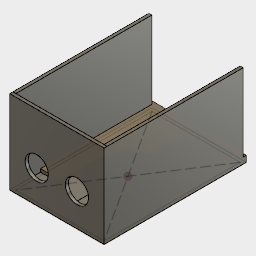
bottom shell v2 v7 (Autodesk Fusion 360 design; units mm, degrees)
Autodesk Fusion 360 part; units mm, degrees
note: some values were not read from the file. Set by a fixed rule: which sketch regions a step uses.
sketch "Sketch1" plane through (0, 0, 0) normal (0, 1, 0) x (1, 0, 0)
  line L0 (14.25, 22) -> (-14.25, 22)
  line L1 (-14.25, 22) -> (-14.25, -22)
  line L2 (-14.25, -22) -> (14.25, -22)
  line L3 (14.25, -22) -> (14.25, 22)
  line L4 (14.25, 22) -> (-14.25, -22) construction
  line L5 (-14.25, 22) -> (14.25, -22) construction
  line L6 (-15.25, 23) -> (-15.25, -23)
  line L7 (-15.25, -23) -> (15.25, -23)
  line L8 (15.25, -23) -> (15.25, 23)
  line L9 (15.25, 23) -> (-15.25, 23)
  dimension "d1" = 44
  dimension "d2" = 28.5
  dimension "d3" = 1
  measures "d1" distance of L0.end L1.end
  measures "d2" distance of L1.end L2.end
extrude "Extrude2" add sketch "Sketch1" along normal blind 2 contours L0 L1 L2 L3 makes body 1
extrude "Extrude1" add sketch "Sketch1" along normal blind 17 separate body makes body 2
sketch "Sketch2" plane through (0, 0, 23) normal (0, 0, 1) x (1, 0, 0)
  line L0 (-15.25, 0) -> (15.25, 0)
  line L1 (15.25, 0) -> (15.25, 17)
  line L2 (15.25, 17) -> (-15.25, 17)
  line L3 (-15.25, 17) -> (-15.25, 0)
  line L4 (0, 0) -> (0, 2)
  line L5 (-14.25, 2) -> (-16.75, 2)
  line L6 (14.25, 2) -> (15.25, 2)
  line L7 (14.25, 0) -> (14.25, 17)
  line L8 (-14.25, 0) -> (-14.25, 17)
  line L9 (-14.25, 2) -> (14.25, 2)
  line L10 (0, 2) -> (0, 4.8)
  line L11 (0, 4.8) -> (0, 8.55)
  line L12 (1.1168, 4.8) -> (-1, 4.8)
  line L13 (14.25, 10.55) -> (10.25, 10.55)
  line L14 (-14.25, 10.55) -> (-10.25, 10.55)
  line L15 (-10.25, 10.55) -> (-6.5, 10.55)
  line L16 (10.25, 10.55) -> (6.5, 10.55)
  circle A0 centre (-6.5, 10.55) radius 3.75
  circle A1 centre (6.5, 10.55) radius 3.75
  line L17 (0, 8.55) -> (0, 10.55)
  line L18 (-14.25, 10.55) -> (-6, 10.55)
  line L19 (14.25, 10.55) -> (6, 10.55)
  point P0 (-14.25, 2)
  point P1 (14.25, 2)
  point P2 (14.25, 0)
  point P3 (14.25, 17)
  point P4 (-14.25, 0)
  point P5 (-14.25, 17)
  dimension "d8" = 2
  dimension "d13" = 2.8
  dimension "d14" = 3.75
  dimension "d15" = 4
  dimension "d16" = 4
  dimension "d17" = 3.75
  dimension "d18" = 3.75
  dimension "d19" = 7.5
  dimension "d20" = 7.5
  dimension "d51" = 2
  measures "d8" distance of L4.start L4.end
  measures "d13" distance of L4.end L10.end
  measures "d14" distance of L10.end L11.end
  measures "d15" distance of L13.start L13.end
  measures "d16" distance of L14.start L14.end
  measures "d17" distance of L14.end L15.end
  measures "d18" distance of L13.end L16.end
  measures "d19" diameter of A0
  measures "d20" diameter of A1
  measures "d51" distance of L11.end L17.end
extrude "Extrude3" cut sketch "Sketch2" against normal blind 6 contours A0 | A1 bodies 2
sketch "Sketch3" plane through (0, 0, -23) normal (0, 0, -1) x (-1, 0, 0)
  line L0 (-15.25, 0) -> (15.25, 0)
  line L1 (15.25, 0) -> (15.25, 17)
  line L2 (15.25, 17) -> (-15.25, 17)
  line L3 (-15.25, 17) -> (-15.25, 0)
  line L4 (0, 0) -> (0, 2)
  line L5 (0, 2) -> (0, 4.8)
  line L6 (0, 4.8) -> (0, 8.55)
  circle A0 centre (0, 8.55) radius 3.75
  dimension "d23" = 2
  dimension "d24" = 2.8
  dimension "d25" = 3.75
  dimension "d26" = 7.5
  measures "d23" distance of L4.start L4.end
  measures "d24" distance of L4.end L5.end
  measures "d25" distance of L5.end L6.end
  measures "d26" diameter of A0
extrude "Extrude4" cut sketch "Sketch3" against normal blind 6 contours A0 bodies 2
sketch "Sketch4" plane through (15.25, 0, 0) normal (1, 0, 0) x (0, 0, -1)
  line L0 (-23, 0) -> (23, 0)
  line L1 (23, 0) -> (23, 17)
  line L2 (23, 17) -> (-23, 17)
  line L3 (-23, 17) -> (-23, 0)
  line L4 (-22, 0) -> (-22, 17)
  line L5 (-23, 4.2398) -> (-22, 4.2398)
  line L6 (23, 4.2398) -> (21.5, 4.2398)
  line L7 (0, 0) -> (0, 2)
  line L8 (-22, 2) -> (22, 2)
  line L9 (22, 2) -> (22, 17)
  line L10 (22, 17) -> (-22, 17)
  line L11 (-22, 17) -> (-22, 2)
  line L12 (-22, 6.4795) -> (22, 6.4795)
  line L13 (22, 6.4795) -> (22, 17)
  line L14 (22, 17) -> (-22, 17)
  line L15 (-22, 17) -> (-22, 6.4795)
  point P0 (-22, 2)
  point P1 (22, 17)
  dimension "d29" = 2
  measures "d29" distance of L7.start L7.end
extrude "Extrude5" cut sketch "Sketch4" against normal blind 71 contours L2 L4 L9 L10 L11 L12 L13 L14 L15 bodies 2
extrude "Extrude6" add 2 faces at (14.9167, 6.4795, 7.3333) (-14.5833, 6.4795, 7.3333) along direction (0, 1, 0) blind 0.02 on bodies 2 bodies 2
extrude "Extrude7" add 1 faces at (-1.71, 2.3531, 22) along direction (0, 0, -1) blind 1 on bodies 2 bodies 2 1
extrude "Extrude8" add 1 faces at (11.0278, 11.0516, -22) along direction (0, 0, 1) blind 1 on bodies 2 bodies 2
sketch "Sketch6" plane through (0, 2, 0) normal (0, 1, 0) x (-1, 0, 0)
  line L0 (-14.25, -21) -> (14.25, -21)
  line L1 (14.25, -21) -> (14.25, 21)
  line L2 (14.25, 21) -> (-14.25, 21)
  line L3 (-14.25, 21) -> (-14.25, -21)
  line L4 (-6, 7) -> (6, 7)
  line L5 (6, 7) -> (6, -7)
  line L6 (6, -7) -> (-6, -7)
  line L7 (-6, -7) -> (-6, 7)
  line L8 (-6, 7) -> (6, -7) construction
  line L9 (6, 7) -> (-6, -7) construction
extrude "Extrude9" cut sketch "Sketch6" against normal blind 1 contours L4 L5 L6 L7 bodies 2
sketch "Sketch7" plane through (0, 2, 0) normal (0, 1, 0) x (-1, 0, 0)
  line L0 (6, 7) -> (6, -7)
  line L1 (6, -7) -> (-6, -7)
  line L2 (-6, -7) -> (-6, 7)
  line L3 (-6, 7) -> (6, 7)
  line L4 (-14.25, -21) -> (14.25, -21)
  line L5 (14.25, -21) -> (14.25, 21)
  line L6 (14.25, 21) -> (-14.25, 21)
  line L7 (-14.25, 21) -> (-14.25, -21)
  line L8 (14.25, 21) -> (-0.75, 21)
  line L9 (-0.75, 21) -> (-0.75, 14)
  line L10 (-0.75, 14) -> (14.25, 14)
  line L11 (14.25, 14) -> (14.25, 21)
  line L12 (-14.25, -21) -> (0.75, -21)
  line L13 (0.75, -21) -> (0.75, -14)
  line L14 (0.75, -14) -> (-14.25, -14)
  line L15 (-14.25, -14) -> (-14.25, -21)
  dimension "d41" = 15
  dimension "d42" = 7
  dimension "d43" = 15
  dimension "d44" = 7
  measures "d41" distance of L9.end L10.end
  measures "d42" distance of L8.end L9.end
  measures "d43" distance of L4.start L12.end
  measures "d44" distance of L4.start L14.end
extrude "Extrude10" cut sketch "Sketch7" against normal blind 1 contours L4 L7 L12 L13 L14 L15 | L5 L6 L8 L9 L10 L11 bodies 2
sketch "Sketch8" plane through (0, 0, -21) normal (0, 0, 1) x (1, 0, 0)
  line L0 (14.25, 1) -> (14.25, 6.4995)
  line L1 (14.25, 6.4995) -> (15.25, 6.4995)
  line L2 (15.25, 6.4995) -> (15.25, 17)
  line L3 (15.25, 17) -> (-15.25, 17)
  line L4 (-15.25, 17) -> (-15.25, 6.4995)
  line L5 (-15.25, 6.4995) -> (-14.25, 6.4995)
  line L6 (-14.25, 6.4995) -> (-14.25, 2)
  line L7 (-14.25, 2) -> (-0.75, 2)
  line L8 (-0.75, 2) -> (-0.75, 1)
  line L9 (-0.75, 1) -> (14.25, 1)
  circle A0 centre (0, 8.55) radius 3.75
  line L10 (-15.25, 17) -> (14.5, 17)
  line L11 (14.5, 17) -> (14.5, 2)
  line L12 (14.5, 2) -> (-15.25, 2)
  line L13 (-15.25, 2) -> (-15.25, 17)
extrude "Extrude11" cut sketch "Sketch8" against normal blind 8 contours L0 L1 L3 L4 L5 L6 L7 L10 L11 L12 L13 | L1 L2 L3 L11 bodies 2
sketch "Sketch9" plane through (0, 0, -23) normal (0, 0, -1) x (-1, 0, 0)
  line L0 (15.25, 6.4995) -> (14.25, 6.4995)
  line L1 (14.25, 6.4995) -> (14.25, 2)
  line L2 (14.25, 2) -> (-14.25, 2)
  line L3 (-14.25, 2) -> (-14.25, 6.4995)
  line L4 (-14.25, 6.4995) -> (-15.25, 6.4995)
  line L5 (-15.25, 6.4995) -> (-15.25, 0)
  line L6 (-15.25, 0) -> (15.25, 0)
  line L7 (15.25, 0) -> (15.25, 6.4995)
  line L8 (14.25, 2) -> (15.25, 1.9841)
  line L9 (-14.25, 2) -> (-14.75, 2)
extrude "Extrude12" cut sketch "Sketch9" against normal blind 2 bodies 2
sketch "Sketch10" plane through (0, 0, -21) normal (0, 0, -1) x (-1, 0, 0)
  line L0 (0.75, 2) -> (0.75, 1)
  line L1 (0.75, 1) -> (-14.25, 1)
  line L2 (-14.25, 1) -> (-14.25, 6.4995)
  line L3 (-14.25, 6.4995) -> (-15.25, 6.4995)
  line L4 (-15.25, 6.4995) -> (-15.25, 0)
  line L5 (-15.25, 0) -> (15.25, 0)
  line L6 (15.25, 0) -> (15.25, 6.4995)
  line L7 (15.25, 6.4995) -> (14.25, 6.4995)
  line L8 (14.25, 6.4995) -> (14.25, 2)
  line L9 (14.25, 2) -> (0.75, 2)
  line L10 (14.25, 2) -> (15.25, 1.9623)
  line L11 (15.25, 2) -> (15.25, 0)
  line L12 (15.25, 0) -> (-15, 0)
  line L13 (14.25, 2) -> (-15.25, 2)
  line L14 (-15.25, 2) -> (15.25, 2)
  line L15 (15.25, 2) -> (15.25, 0)
  line L16 (15.25, 0) -> (-15.25, 0)
  line L17 (-15.25, 0) -> (-15.25, 2)
  point P0 (-14.25, 2)
extrude "Extrude13" add sketch "Sketch10" along normal blind 1 contours L6 L7 L8 L14 | L2 L3 L4 L13 L14 bodies 2
extrude "Extrude14" add 1 faces at (-10.0833, 1, -21) along direction (0, 0, -1) blind 2 on bodies 2 bodies 2
sketch "Sketch11" plane through (14.25, 0, 0) normal (-1, 0, 0) x (0, 0, 1)
  line L0 (-23, 1) -> (-14, 1)
  line L1 (-14, 1) -> (-14, 2)
  line L2 (-14, 2) -> (21, 2)
  line L3 (21, 2) -> (21, 6.4995)
  line L4 (21, 6.4995) -> (-22, 6.4995)
  line L5 (-22, 6.4995) -> (-22, 2)
  line L6 (-22, 2) -> (-23, 2)
  line L7 (-23, 2) -> (-23, 1)
  line L8 (-22, 2) -> (-22, 1)
extrude "Extrude15" add sketch "Sketch11" along normal blind 15 contours L0 L6 L7 L8 bodies 2
extrude "Extrude16" cut 1 faces at (-6.7601, 2.9368, 21) along direction (0, 0, 1) blind 1 on bodies 2 bodies 2
sketch "Sketch12" plane through (0, 2, 0) normal (0, 1, 0) x (-1, 0, 0)
  line L0 (6, 7) -> (6, -7)
  line L1 (6, -7) -> (-6, -7)
  line L2 (-6, -7) -> (-6, 7)
  line L3 (-6, 7) -> (6, 7)
  line L4 (-14.25, -22) -> (-15.25, -22)
  line L5 (-15.25, -22) -> (-15.25, -23)
  line L6 (-15.25, -23) -> (15.25, -23)
  line L7 (15.25, -23) -> (15.25, -22)
  line L8 (15.25, -22) -> (14.25, -22)
  line L9 (14.25, -22) -> (14.25, 14)
  line L10 (14.25, 14) -> (-0.75, 14)
  line L11 (-0.75, 14) -> (-0.75, 22)
  line L12 (-0.75, 22) -> (-14.25, 22)
  line L13 (-14.25, 22) -> (-14.25, -14)
  line L14 (-14.25, -14) -> (0.75, -14)
  line L15 (0.75, -14) -> (0.75, -22)
  line L16 (0.75, -22) -> (-14.25, -22)
  line L17 (0.75, -14) -> (-8, -14)
  line L18 (-8, -14) -> (-8, 0)
  line L19 (-8, 0) -> (0.75, 0)
  line L20 (0.75, 0) -> (0.75, -14)
extrude "Extrude17" cut sketch "Sketch12" against normal blind 1 contours L1 L2 L14 L17 L18 L19 L20 | L1 L2 L19 L20 bodies 2
sketch "Sketch13" plane through (0, 2, 0) normal (0, 1, 0) x (-1, 0, 0)
  line L0 (0.75, -7) -> (0.75, -22)
  line L1 (0.75, -22) -> (-14.25, -22)
  line L2 (-14.25, -22) -> (-15.25, -22)
  line L3 (-15.25, -22) -> (-15.25, -23)
  line L4 (-15.25, -23) -> (15.25, -23)
  line L5 (15.25, -23) -> (15.25, -22)
  line L6 (15.25, -22) -> (14.25, -22)
  line L7 (14.25, -22) -> (14.25, 14)
  line L8 (14.25, 14) -> (-0.75, 14)
  line L9 (-0.75, 14) -> (-0.75, 22)
  line L10 (-0.75, 22) -> (-14.25, 22)
  line L11 (-14.25, 22) -> (-14.25, -14)
  line L12 (-14.25, -14) -> (-8, -14)
  line L13 (-8, -14) -> (-8, 0)
  line L14 (-8, 0) -> (-6, 0)
  line L15 (-6, 0) -> (-6, 7)
  line L16 (-6, 7) -> (6, 7)
  line L17 (6, 7) -> (6, -7)
  line L18 (6, -7) -> (0.75, -7)
  line L19 (-0.75, 14) -> (8, 14)
  line L20 (8, 14) -> (8, 0)
  line L21 (8, 0) -> (-0.75, 0)
  line L22 (-0.75, 0) -> (-0.75, 14)
extrude "Extrude18" cut sketch "Sketch13" against normal blind 1 contours L8 L16 L17 L19 L20 L21 L22 bodies 2
extrude "Extrude19" add 1 faces at (5.0833, 17, 22.6667) along direction (0, 1, 0) blind 10 on bodies 2 bodies 2
extrude "Extrude20" add 2 faces at (-14.9167, 6.4995, 7.3333) (14.9167, 6.4995, -7.3333) along direction (0, 1, 0) blind 20.5 on bodies 2 bodies 2
sketch "Sketch14" plane through (0, 2, 0) normal (0, 1, 0) x (-1, 0, 0)
  line L0 (8, 14) -> (8, 0)
  line L1 (8, 0) -> (6, 0)
  line L2 (6, 0) -> (6, -7)
  line L3 (6, -7) -> (0.75, -7)
  line L4 (0.75, -7) -> (0.75, -22)
  line L5 (0.75, -22) -> (-14.25, -22)
  line L6 (-14.25, -22) -> (-15.25, -22)
  line L7 (-15.25, -22) -> (-15.25, -23)
  line L8 (-15.25, -23) -> (15.25, -23)
  line L9 (15.25, -23) -> (15.25, -22)
  line L10 (15.25, -22) -> (14.25, -22)
  line L11 (14.25, -22) -> (14.25, 14)
  line L12 (14.25, 14) -> (8, 14)
equation "d14 = ( 7.5 / 2 ) * 1 mm"
equation "d17 = ( 7.5 / 2 ) * 1 mm"
equation "d18 = ( 7.5 / 2 ) * 1 mm"
equation "d25 = ( 7.5 / 2 ) * 1 mm"
